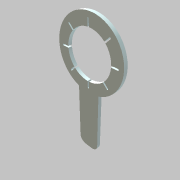
# Autodesk Inventor part: Mutternschlüssel
Saved by Autodesk Inventor 2015 (Build 190159000, 159)
## iProperties
Created: 2016-09-04
Part Number: Mutternschlüssel
Material: Generic
Document SubType Name: Modeling
Designer: Seelenernter
Density: 1 g/cm^3
Appearance: Default
Author: Seelenernter
Autodesk Inventor part; units mm, degrees
ref_plane "YZ Plane" through (0, 0, 0) normal (1, 0, 0) x (0, 1, 0)
ref_plane "XZ Plane" through (0, 0, 0) normal (0, 1, 0) x (-1, 0, 0)
ref_plane "XY Plane" through (0, 0, 0) normal (0, 0, 1) x (1, 0, 0)
sketch "Skizze1" plane through (0, 0, 0) normal (0, 1, 0) x (-1, 0, 0)
  line L0 (0, -165) -> (0, 80) projected
  line L1 (-63, 0) -> (63, 0) projected
  line L2 (63, 0) -> (-63, 0) projected
  line L3 (0, -165) -> (0, 80) projected
  circle A0 centre (0, 0) radius 30
  circle A1 centre (0, 0) radius 45
  line L4 (15, -42.4264) -> (15, -130)
  line L5 (15, -130) -> (-15, -130)
  line L6 (-15, -130) -> (-15, -42.4264)
  dimension "d0" = 60
  dimension "d1" = 90
  dimension "d2" = 30
  dimension "d3" = 15
  dimension "d4" = 130
  constraints: 6 end point, 2 centre point, 2 coincident, 2 perpendicular, 2 point on circle, 1 vertical
  measures "d0" diameter of A0
  measures "d1" diameter of A1
  measures "d2" distance of L4.end L5.end
  measures "d3" distance between parallel lines of L0 L6
  measures "d4" distance between parallel lines of L1 L5
extrude "Extrusion1" add sketch "Skizze1" along normal blind 5 contours L5 L6 A1 L0 | L0 A1 L4 L5 | A1 L1 A0 L0 | L0 A0 L1 A1 | L1 A1 L0 A0 | A0 L0 A1 L1
fillet "Rundung1" radius 10 2 edges at (-15, 2.5, -130) (15, 2.5, -130)
sketch "Skizze2" plane through (0, 5, 0) normal (0, 1, 0) x (1, 0, 0)
  line L0 (0, 167.4853) -> (0, -80.4142) projected
  line L1 (63, 0) -> (-63, 0) projected
  line L2 (-63, 0) -> (63, 0) projected
  arc A0 (15, 120) -> (5, 130) centre (5, 120) ccw projected
  line L3 (-15, 120) -> (-15, 42.4264) projected
  arc A1 (-15, 42.4264) -> (15, 42.4264) centre (0, 0) ccw projected
  line L4 (15, 42.4264) -> (15, 120) projected
  circle A2 centre (0, 0) radius 30 projected
  circle A3 centre (0, 0) radius 30
  circle A4 centre (0, 0) radius 30 projected
  line L5 (1, -29.9833) -> (1, -39)
  line L6 (1, -39) -> (-1, -39)
  line L7 (-1, -39) -> (-1, -29.9833)
  line L8 (5, 130) -> (-5, 130) projected
  arc A5 (-5, 130) -> (-15, 120) centre (-5, 120) ccw projected
  dimension "d8" = 1
  dimension "d9" = 2
  dimension "d10" = 9
  constraints: 6 end point, 2 perpendicular, 2 point on circle, 1 coincident, 1 vertical, 3 other
  measures "d8" distance between parallel lines of L0 L5
  measures "d9" distance of L5.end L6.end
  measures "d10" distance edge to line of A2 L6
extrude "Extrusion2" cut sketch "Skizze2" against normal blind 5 contours A2 L5 L6 L0 | L0 L6 L7 A2
fillet "Rundung2" radius 1 2 edges at (-1, 2.5, 39) (1, 2.5, 39)
pattern_circular "Runde Anordnung1" count 8 over 360 about axis through (0, 0, 0) along (0, 1, 0) of "Rundung2", "Extrusion2"
